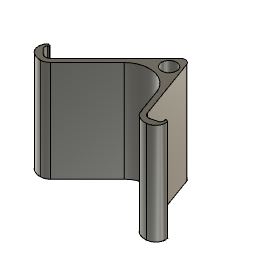
iPad Stand (Autodesk Fusion 360 design; units mm, degrees)
Autodesk Fusion 360 part; units mm, degrees
sketch "Sketch1" plane through (0, 0, 0) normal (0, 0, 1) x (1, 0, 0)
  line L0 (3.5355, 3.5355) -> (67.7657, 67.7657)
  line L1 (98.2899, 4.6985) -> (75.9997, 65.9403)
  line L2 (-3.5355, 3.5355) -> (-8.4853, 8.4853)
  arc A0 (75.9997, 65.9403) -> (67.7657, 67.7657) centre (71.3012, 64.2302) ccw
  line L3 (-8.4853, 12.7279) -> (-7.6674, 13.5458)
  line L4 (-10.6066, 10.6066) -> (-5.6066, 10.6066) construction
  arc A1 (-3.5355, 3.5355) -> (3.5355, 3.5355) centre (0, 7.0711) ccw
  arc A2 (-8.4853, 12.7279) -> (-8.4853, 8.4853) centre (-6.364, 10.6066) ccw
  line L5 (7.0711, 0) -> (43.5529, 36.4818)
  line L6 (93.5914, 2.9884) -> (84.7228, 27.3546)
  arc A3 (84.7228, 27.3546) -> (43.5529, 36.4818) centre (61.2305, 18.8041) ccw
  circle A4 centre (69.2871, 55.145) radius 7.5
  arc A5 (0, -2.9289) -> (7.0711, 0) centre (0, 7.0711) ccw
  line L7 (0, -2.9289) -> (0, -2.9289)
  line L8 (-9.9476, 15.0524) -> (-10, 15)
  line L9 (-9.405, 14.8257) -> (-7.8804, 14.3792)
  arc A6 (-8.6295, -0.1981) -> (0, -2.9289) centre (0, 12.0711) ccw
  arc A7 (-10.4427, 14.5199) -> (-8.6295, -0.1981) centre (-2.8765, 7.9814) ccw
  arc A8 (-9.405, 14.8257) -> (-10.4427, 14.5199) centre (-9.6861, 13.866) ccw
  arc A9 (-7.6674, 13.5458) -> (-7.8804, 14.3792) centre (-8.021, 13.8993) ccw
  arc A10 (111.0144, 2.9071) -> (113.1357, 6.5813) centre (110.2379, 5.8048) ccw
  line L10 (97.9588, -2.7353) -> (97.9588, -2.7353)
  arc A11 (98.2899, 4.6985) -> (104.3967, 1.1339) centre (103.1256, 5.9696) ccw
  line L11 (115.5643, 7.8632) -> (115.5835, 7.7916)
  arc A12 (113.4375, 8.3138) -> (112.8363, 7.6985) centre (113.3193, 7.8279) ccw
  line L12 (104.3967, 1.1339) -> (111.0144, 2.9071)
  arc A13 (115.7269, 7.1545) -> (114.9811, 7.9382) centre (114.7447, 6.9665) ccw
  line L13 (113.1357, 6.5813) -> (112.8363, 7.6985)
  arc A14 (106.7976, -4.6851) -> (115.7269, 7.1545) centre (105.9051, 5.275) ccw
  line L14 (114.9811, 7.9382) -> (113.4375, 8.3138)
  arc A15 (93.5914, 2.9884) -> (97.9588, -2.7353) centre (103.1064, 5.7205) ccw
  arc A16 (97.9588, -2.7353) -> (106.7976, -4.6851) centre (105.4588, 10.2551) ccw
  point P0 (100, 0)
  point P1 (-7.0711, 14.1421)
  point P2 (95.6559, -0.9674)
  point P3 (102.727, -0.9674)
  point P4 (99.4233, -0.1988)
  point P5 (112.6181, 8.5131)
  dimension "d2" = 100
  dimension "d6" = 15
  dimension "d9" = 5
  dimension "d10" = 45
  dimension "d11" = 5
  dimension "d13" = 5
  dimension "d15" = 3
  dimension "d19" = 25
  dimension "d20" = 15
  dimension "d21" = 10
  dimension "d23" = 10
  dimension "d26" = 15
  dimension "d27" = 10
  dimension "d28" = 1
  dimension "d29" = 0.5
  constraint perpendicular L0 L2
  constraint tangent L0 A0
  constraint tangent L1 A0
  constraint horizontal L4
  constraint perpendicular L2 L3
  constraint coincident origin L0
  constraint coincident origin L2
  constraint tangent L0 A1
  constraint tangent L2 A1
  constraint coincident P0 L1
  constraint coincident L4.start L3
  constraint coincident L4.start L2
  constraint tangent L3 A2
  constraint tangent L2 A2
  constraint parallel L0 L5
  constraint parallel L1 L6
  constraint tangent L5 A3
  constraint tangent L6 A3
  constraint concentric A1 A5
  constraint tangent A6 A7
  constraint tangent L8 A7
  constraint tangent A7 A8
  constraint tangent L9 A8
  constraint coincident P1 L9
  constraint coincident P1 L3
  constraint tangent L9 A9
  constraint tangent L3 A9
  constraint coincident L6.start A15.start
  constraint coincident L1.start A11.start
  measures "d2" distance of origin P0
  measures "d6" distance of origin L4.start
  measures "d9" radius of A0
  measures "d10" angle of L3 L4
  measures "d11" distance of L4.start P1
  measures "d13" radius of A1
  measures "d15" radius of A2
  measures "d19" radius of A3
  measures "d20" diameter of A4
  measures "d21" distance of L0 A4.centre
  measures "d23" distance of L1 A4.centre
  measures "d26" radius of A6
  measures "d27" radius of A7
  measures "d28" radius of A8
  measures "d29" radius of A9
extrude "Extrude1" add sketch "Sketch1" along normal blind 100
sketch "Sketch2" plane through (0, 0, 0) normal (-0.707107, 0.707107, 0) x (-0.707107, -0.707107, 0)
  line L0 (-95.8352, 0) -> (-5, 0)
  line L1 (-5, 0) -> (-5, 100)
  line L2 (-5, 100) -> (-95.8352, 100)
  line L3 (-95.8352, 100) -> (-95.8352, 0)
  ellipse E0 centre (-30, 50) end of major axis (-30, 90) minor radius 20
  line L4 (-30, 10) -> (-30, 90)
  line L5 (-10, 50) -> (-50, 50)
  constraint vertical L4
  constraint coincident E0 L4.start
  constraint coincident E0 L4.end
  constraint coincident E0 L5.start
  constraint coincident E0 L5.end
sketch "Sketch3" plane through (88.3022, 32.1394, 0) normal (0.939693, 0.34202, 0) x (-0.34202, 0.939693, 0)
  line L0 (-29.202, 0) -> (35.9702, 0)
  line L1 (35.9702, 0) -> (35.9702, 100)
  line L2 (35.9702, 100) -> (-29.202, 100)
  line L3 (-29.202, 100) -> (-29.202, 0)
  ellipse E0 centre (-15, 50) end of major axis (-15, 90) minor radius 10
  line L4 (-15, 10) -> (-15, 90)
  line L5 (-5, 50) -> (-25, 50)
  dimension "d35" = 20
  constraint vertical L4
  constraint coincident E0 L4.start
  constraint coincident E0 L4.end
  constraint coincident E0 L5.start
  constraint coincident E0 L5.end
extrude "Extrude3" [suppressed]
extrude "Extrude4" [suppressed]
